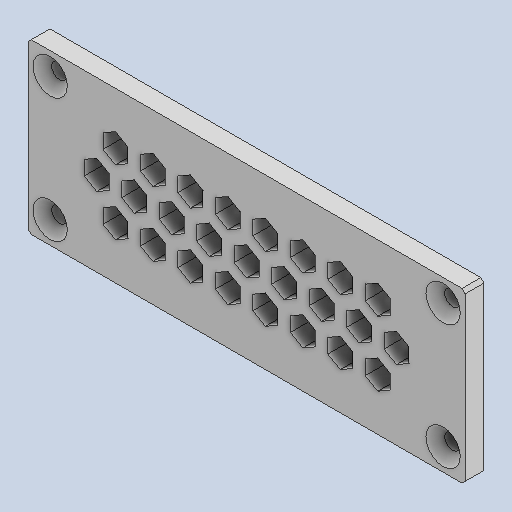
# Autodesk Inventor part: A-04
Saved by Autodesk Inventor 2022.2 (Build 262287000, 287)
## iProperties
Created: 2021-12-13
Part Number: A-04
Material: Generic
Document SubType Name: Modeling
Designer: kfcs7
Density: 1 g/cm^3
Appearance: Default
Author: kfcs7
Autodesk Inventor part; units mm, degrees
ref_plane "YZ Plane" through (0, 0, 0) normal (1, 0, 0) x (0, 1, 0)
ref_plane "XZ Plane" through (0, 0, 0) normal (0, 1, 0) x (-1, 0, 0)
ref_plane "XY Plane" through (0, 0, 0) normal (0, 0, 1) x (1, 0, 0)
sketch "Sketch1" plane through (0, 0, 0) normal (0, 0, 1) x (1, 0, 0)
  circle A0 centre (66.4645, 3.5355) radius 2 construction
  line L0 (0.5, 0) -> (0, 0.5) projected
  line L1 (0.5, 0) -> (69.5, 0) projected
  line L2 (70, 0.5) -> (69.5, 0) projected
  line L3 (70, 0.5) -> (70, 9.5) construction
  line L4 (70, 9.5) -> (67, 9.5) construction
  line L5 (67, 17.5) -> (67, 9.5) construction
  line L6 (65, 17.5) -> (67, 17.5) construction
  line L7 (65, 17.5) -> (65, 8.0711) construction
  line L8 (65, 8.0711) -> (61.9289, 5) construction
  line L9 (61.9289, 5) -> (8.0711, 5) construction
  line L10 (8.0711, 5) -> (5, 8.0711) construction
  line L11 (5, 8.0711) -> (5, 17.5) construction
  line L12 (3, 17.5) -> (5, 17.5) construction
  line L13 (3, 9.5) -> (3, 17.5) construction
  line L14 (3, 9.5) -> (0, 9.5) construction
  line L15 (0, 0.5) -> (0, 9.5) construction
  circle A1 centre (3.5355, 3.5355) radius 2 construction
  circle A2 centre (3.5355, 23.4645) radius 2 construction
  circle A3 centre (66.4645, 23.4645) radius 2 construction
  line L16 (65, 17.5) -> (67.5, 17.5) construction
  line L17 (67.5, 17.5) -> (67.5, 9.5) construction
  line L18 (70, 9.5) -> (67.5, 9.5) construction
  line L19 (70, 26.5) -> (70, 9.5) construction
  line L20 (69.5, 27) -> (70, 26.5) projected
  line L21 (69.5, 27) -> (0.5, 27) projected
  line L22 (0, 26.5) -> (0.5, 27) projected
  line L23 (0, 26.5) -> (0, 9.5) construction
  line L24 (2.5, 9.5) -> (0, 9.5) construction
  line L25 (2.5, 9.5) -> (2.5, 17.5) construction
  line L26 (2.5, 17.5) -> (5, 17.5) construction
  line L27 (5, 17.5) -> (5, 18.9289) construction
  line L28 (5, 18.9289) -> (8.0711, 22) construction
  line L29 (8.0711, 22) -> (61.9289, 22) construction
  line L30 (61.9289, 22) -> (65, 18.9289) construction
  line L31 (65, 18.9289) -> (65, 17.5) construction
  line L32 (70, 26.5) -> (70, 0.5)
  line L33 (0, 0.5) -> (0, 26.5)
  point P0 (0, 0)
  constraints: 4 end point, 2 collinear
extrude "Extrusion1" add sketch "Sketch1" along normal blind 3
sketch "Sketch2" plane through (0, 0, 3) normal (0, 0, 1) x (1, 0, 0)
  circle A0 centre (3.5355, 23.4645) radius 2 construction
  circle A1 centre (66.4645, 23.4645) radius 2 construction
  line L0 (65, 17.5) -> (67.5, 17.5) construction
  line L1 (67.5, 17.5) -> (67.5, 9.5) construction
  line L2 (70, 9.5) -> (67.5, 9.5) construction
  line L3 (70, 26.5) -> (70, 9.5) construction
  line L4 (69.5, 27) -> (70, 26.5) construction
  line L5 (69.5, 27) -> (0.5, 27) construction
  line L6 (0, 26.5) -> (0.5, 27) construction
  line L7 (0, 26.5) -> (0, 9.5) construction
  line L8 (2.5, 9.5) -> (0, 9.5) construction
  line L9 (2.5, 9.5) -> (2.5, 17.5) construction
  line L10 (2.5, 17.5) -> (5, 17.5) construction
  line L11 (5, 17.5) -> (5, 18.9289) construction
  line L12 (5, 18.9289) -> (8.0711, 22) construction
  line L13 (8.0711, 22) -> (61.9289, 22) construction
  line L14 (61.9289, 22) -> (65, 18.9289) construction
  line L15 (65, 18.9289) -> (65, 17.5) construction
  circle A2 centre (66.4645, 3.5355) radius 2 construction
  line L16 (0.5, 0) -> (0, 0.5) construction
  line L17 (0.5, 0) -> (69.5, 0) construction
  line L18 (70, 0.5) -> (69.5, 0) construction
  line L19 (70, 0.5) -> (70, 9.5) construction
  line L20 (70, 9.5) -> (67, 9.5) construction
  line L21 (67, 17.5) -> (67, 9.5) construction
  line L22 (65, 17.5) -> (67, 17.5) construction
  line L23 (65, 17.5) -> (65, 8.0711) construction
  line L24 (65, 8.0711) -> (61.9289, 5) construction
  line L25 (61.9289, 5) -> (8.0711, 5) construction
  line L26 (8.0711, 5) -> (5, 8.0711) construction
  line L27 (5, 8.0711) -> (5, 17.5) construction
  line L28 (3, 17.5) -> (5, 17.5) construction
  line L29 (3, 9.5) -> (3, 17.5) construction
  line L30 (3, 9.5) -> (0, 9.5) construction
  line L31 (0, 0.5) -> (0, 9.5) construction
  circle A3 centre (3.5355, 3.5355) radius 2 construction
  circle A4 centre (3.5355, 23.4645) radius 1.25
  circle A5 centre (3.5355, 3.5355) radius 1.25
  circle A6 centre (66.4645, 3.5355) radius 1.25
  circle A7 centre (66.4645, 23.4645) radius 1.25
  point P0 (0, 0)
  dimension "d2" = 2.5
  dimension "d3" = 2.5
  dimension "d4" = 2.5
  dimension "d5" = 2.5
  constraints: 4 centre point, 4 coincident
  measures "d2" diameter of A4
  measures "d3" diameter of A5
  measures "d4" diameter of A6
  measures "d5" diameter of A7
extrude "Extrusion2" cut sketch "Sketch2" against normal through all
chamfer "Chamfer1" distance 1.5 angle 45 4 edges at (2.2855, 23.4645, 3) (2.2855, 3.5355, 3) (65.2145, 3.5355, 3) (65.2145, 23.4645, 3)
sketch "Sketch3" plane through (0, 0, 3) normal (0, 0, 1) x (1, 0, 0)
  circle A0 centre (66.4645, 3.5355) radius 2.75 projected
  circle A1 centre (3.5355, 23.4645) radius 2.75 projected
  line L0 (0.5, 27) -> (0, 26.5) projected
  line L1 (0, 26.5) -> (0, 0.5) projected
  line L2 (0, 0.5) -> (0.5, 0) projected
  line L3 (0.5, 0) -> (69.5, 0) projected
  line L4 (69.5, 0) -> (70, 0.5) projected
  line L5 (70, 0.5) -> (70, 26.5) projected
  line L6 (70, 26.5) -> (69.5, 27) projected
  line L7 (69.5, 27) -> (0.5, 27) projected
  circle A2 centre (3.5355, 3.5355) radius 2.75 projected
  circle A3 centre (66.4645, 23.4645) radius 2.75 projected
  line L8 (32, 15.2321) -> (35, 16.9641)
  line L9 (35, 16.9641) -> (38, 15.2321)
  line L10 (38, 15.2321) -> (38, 11.7679)
  line L11 (38, 11.7679) -> (35, 10.0359)
  line L12 (35, 10.0359) -> (32, 11.7679)
  line L13 (32, 11.7679) -> (32, 15.2321)
  line L14 (69.5, 27) -> (0.5, 27) projected
  line L15 (35, 15.8094) -> (33, 14.6547)
  line L16 (33, 14.6547) -> (33, 12.3453)
  line L17 (33, 12.3453) -> (35, 11.1906)
  line L18 (35, 11.1906) -> (37, 12.3453)
  line L19 (37, 12.3453) -> (37, 14.6547)
  line L20 (37, 14.6547) -> (35, 15.8094)
  line L21 (35, 16.9641) -> (35, 20.4282)
  line L22 (35, 20.4282) -> (32, 22.1603)
  line L23 (32, 22.1603) -> (29, 20.4282)
  line L24 (29, 20.4282) -> (29, 16.9641)
  line L25 (29, 16.9641) -> (32, 15.2321)
  line L26 (34, 17.5415) -> (32, 16.3868)
  line L27 (32, 16.3868) -> (30, 17.5415)
  line L28 (30, 17.5415) -> (30, 19.8509)
  line L29 (30, 19.8509) -> (32, 21.0056)
  line L30 (32, 21.0056) -> (34, 19.8509)
  line L31 (34, 19.8509) -> (34, 17.5415)
  line L32 (38, 4.8397) -> (41, 6.5718)
  line L33 (41, 6.5718) -> (41, 10.0359)
  line L34 (41, 10.0359) -> (38, 11.7679)
  line L35 (35, 10.0359) -> (35, 6.5718)
  line L36 (35, 6.5718) -> (38, 4.8397)
  line L37 (40, 7.1491) -> (38, 5.9944)
  line L38 (38, 5.9944) -> (36, 7.1491)
  line L39 (36, 7.1491) -> (36, 9.4585)
  line L40 (36, 9.4585) -> (38, 10.6132)
  line L41 (38, 10.6132) -> (40, 9.4585)
  line L42 (40, 9.4585) -> (40, 7.1491)
  point P0 (0, 0)
  point P1 (35, 13.5)
  point P2 (32, 18.6962)
  point P3 (38, 8.3038)
  dimension "d12" = 27
  dimension "d13" = 13.5
  dimension "d14" = 35
  dimension "d15" = 70
  dimension "d16" = 6
  dimension "d19" = 1
  constraints: 68 end point, 22 symmetric about line, 1 perpendicular, 18 other
  measures "d12" distance between parallel lines of L7 L3
  measures "d13" distance from line of L3 point (35, 13.5)
  measures "d14" distance from line of L5 point (35, 13.5)
  measures "d15" distance between parallel lines of L5 L1
  measures "d16" distance between parallel lines of L10 L13
  measures "d19" distance between parallel lines of L8 L15
extrude "Extrusion3" cut sketch "Sketch3" against normal through all contours L20 L19 L18 L17 L16 L15 | L26 L27 L28 L29 L30 L31 | L37 L38 L39 L40 L41 L42
pattern_linear "Rectangular Pattern1" count 9 spacing 6 along (-1, 0, 0) of "Extrusion3" first direction both ways yes
sketch "Sketch4" plane through (0, 0, 3) normal (0, 0, 1) x (1, 0, 0)
  line L0 (16, 7.1491) -> (14, 5.9944) projected
  line L1 (14, 5.9944) -> (12, 7.1491) projected
  line L2 (12, 7.1491) -> (12, 9.4585) projected
  line L3 (12, 9.4585) -> (14, 10.6132) projected
  line L4 (14, 10.6132) -> (16, 9.4585) projected
  line L5 (16, 9.4585) -> (16, 7.1491) projected
  line L6 (11, 15.8094) -> (13, 14.6547) projected
  line L7 (13, 14.6547) -> (13, 12.3453) projected
  line L8 (13, 12.3453) -> (11, 11.1906) projected
  line L9 (11, 11.1906) -> (9, 12.3453) projected
  line L10 (9, 12.3453) -> (9, 14.6547) projected
  line L11 (9, 14.6547) -> (11, 15.8094) projected
  line L12 (6, 17.5415) -> (6, 19.8509) projected
  line L13 (6, 19.8509) -> (8, 21.0056) projected
  line L14 (8, 21.0056) -> (10, 19.8509) projected
  line L15 (10, 19.8509) -> (10, 17.5415) projected
  line L16 (10, 17.5415) -> (8, 16.3868) projected
  line L17 (8, 16.3868) -> (6, 17.5415) projected
  line L18 (22, 7.1491) -> (20, 5.9944) projected
  line L19 (20, 5.9944) -> (18, 7.1491) projected
  line L20 (18, 7.1491) -> (18, 9.4585) projected
  line L21 (18, 9.4585) -> (20, 10.6132) projected
  line L22 (20, 10.6132) -> (22, 9.4585) projected
  line L23 (22, 9.4585) -> (22, 7.1491) projected
  line L24 (17, 15.8094) -> (19, 14.6547) projected
  line L25 (19, 14.6547) -> (19, 12.3453) projected
  line L26 (19, 12.3453) -> (17, 11.1906) projected
  line L27 (17, 11.1906) -> (15, 12.3453) projected
  line L28 (15, 12.3453) -> (15, 14.6547) projected
  line L29 (15, 14.6547) -> (17, 15.8094) projected
  line L30 (12, 17.5415) -> (12, 19.8509) projected
  line L31 (12, 19.8509) -> (14, 21.0056) projected
  line L32 (14, 21.0056) -> (16, 19.8509) projected
  line L33 (16, 19.8509) -> (16, 17.5415) projected
  line L34 (16, 17.5415) -> (14, 16.3868) projected
  line L35 (14, 16.3868) -> (12, 17.5415) projected
  line L36 (28, 7.1491) -> (26, 5.9944) projected
  line L37 (26, 5.9944) -> (24, 7.1491) projected
  line L38 (24, 7.1491) -> (24, 9.4585) projected
  line L39 (24, 9.4585) -> (26, 10.6132) projected
  line L40 (26, 10.6132) -> (28, 9.4585) projected
  line L41 (28, 9.4585) -> (28, 7.1491) projected
  line L42 (23, 15.8094) -> (25, 14.6547) projected
  line L43 (25, 14.6547) -> (25, 12.3453) projected
  line L44 (25, 12.3453) -> (23, 11.1906) projected
  line L45 (23, 11.1906) -> (21, 12.3453) projected
  line L46 (21, 12.3453) -> (21, 14.6547) projected
  line L47 (21, 14.6547) -> (23, 15.8094) projected
  line L48 (18, 17.5415) -> (18, 19.8509) projected
  line L49 (18, 19.8509) -> (20, 21.0056) projected
  line L50 (20, 21.0056) -> (22, 19.8509) projected
  line L51 (22, 19.8509) -> (22, 17.5415) projected
  line L52 (22, 17.5415) -> (20, 16.3868) projected
  line L53 (20, 16.3868) -> (18, 17.5415) projected
  line L54 (34, 7.1491) -> (32, 5.9944) projected
  line L55 (32, 5.9944) -> (30, 7.1491) projected
  line L56 (30, 7.1491) -> (30, 9.4585) projected
  line L57 (30, 9.4585) -> (32, 10.6132) projected
  line L58 (32, 10.6132) -> (34, 9.4585) projected
  line L59 (34, 9.4585) -> (34, 7.1491) projected
  line L60 (29, 15.8094) -> (31, 14.6547) projected
  line L61 (31, 14.6547) -> (31, 12.3453) projected
  line L62 (31, 12.3453) -> (29, 11.1906) projected
  line L63 (29, 11.1906) -> (27, 12.3453) projected
  line L64 (27, 12.3453) -> (27, 14.6547) projected
  line L65 (27, 14.6547) -> (29, 15.8094) projected
  line L66 (24, 17.5415) -> (24, 19.8509) projected
  line L67 (24, 19.8509) -> (26, 21.0056) projected
  line L68 (26, 21.0056) -> (28, 19.8509) projected
  line L69 (28, 19.8509) -> (28, 17.5415) projected
  line L70 (28, 17.5415) -> (26, 16.3868) projected
  line L71 (26, 16.3868) -> (24, 17.5415) projected
  line L72 (46, 7.1491) -> (44, 5.9944) projected
  line L73 (44, 5.9944) -> (42, 7.1491) projected
  line L74 (42, 7.1491) -> (42, 9.4585) projected
  line L75 (42, 9.4585) -> (44, 10.6132) projected
  line L76 (44, 10.6132) -> (46, 9.4585) projected
  line L77 (46, 9.4585) -> (46, 7.1491) projected
  line L78 (41, 15.8094) -> (43, 14.6547) projected
  line L79 (43, 14.6547) -> (43, 12.3453) projected
  line L80 (43, 12.3453) -> (41, 11.1906) projected
  line L81 (41, 11.1906) -> (39, 12.3453) projected
  line L82 (39, 12.3453) -> (39, 14.6547) projected
  line L83 (39, 14.6547) -> (41, 15.8094) projected
  line L84 (36, 17.5415) -> (36, 19.8509) projected
  line L85 (36, 19.8509) -> (38, 21.0056) projected
  line L86 (38, 21.0056) -> (40, 19.8509) projected
  line L87 (40, 19.8509) -> (40, 17.5415) projected
  line L88 (40, 17.5415) -> (38, 16.3868) projected
  line L89 (38, 16.3868) -> (36, 17.5415) projected
  line L90 (52, 7.1491) -> (50, 5.9944) projected
  line L91 (50, 5.9944) -> (48, 7.1491) projected
  line L92 (48, 7.1491) -> (48, 9.4585) projected
  line L93 (48, 9.4585) -> (50, 10.6132) projected
  line L94 (50, 10.6132) -> (52, 9.4585) projected
  line L95 (52, 9.4585) -> (52, 7.1491) projected
  line L96 (47, 15.8094) -> (49, 14.6547) projected
  line L97 (49, 14.6547) -> (49, 12.3453) projected
  line L98 (49, 12.3453) -> (47, 11.1906) projected
  line L99 (47, 11.1906) -> (45, 12.3453) projected
  line L100 (45, 12.3453) -> (45, 14.6547) projected
  line L101 (45, 14.6547) -> (47, 15.8094) projected
  line L102 (42, 17.5415) -> (42, 19.8509) projected
  line L103 (42, 19.8509) -> (44, 21.0056) projected
  line L104 (44, 21.0056) -> (46, 19.8509) projected
  line L105 (46, 19.8509) -> (46, 17.5415) projected
  line L106 (46, 17.5415) -> (44, 16.3868) projected
  line L107 (44, 16.3868) -> (42, 17.5415) projected
  line L108 (58, 7.1491) -> (56, 5.9944) projected
  line L109 (56, 5.9944) -> (54, 7.1491) projected
  line L110 (54, 7.1491) -> (54, 9.4585) projected
  line L111 (54, 9.4585) -> (56, 10.6132) projected
  line L112 (56, 10.6132) -> (58, 9.4585) projected
  line L113 (58, 9.4585) -> (58, 7.1491) projected
  line L114 (53, 15.8094) -> (55, 14.6547) projected
  line L115 (55, 14.6547) -> (55, 12.3453) projected
  line L116 (55, 12.3453) -> (53, 11.1906) projected
  line L117 (53, 11.1906) -> (51, 12.3453) projected
  line L118 (51, 12.3453) -> (51, 14.6547) projected
  line L119 (51, 14.6547) -> (53, 15.8094) projected
  line L120 (48, 17.5415) -> (48, 19.8509) projected
  line L121 (48, 19.8509) -> (50, 21.0056) projected
  line L122 (50, 21.0056) -> (52, 19.8509) projected
  line L123 (52, 19.8509) -> (52, 17.5415) projected
  line L124 (52, 17.5415) -> (50, 16.3868) projected
  line L125 (50, 16.3868) -> (48, 17.5415) projected
  line L126 (64, 7.1491) -> (62, 5.9944) projected
  line L127 (62, 5.9944) -> (60, 7.1491) projected
  line L128 (60, 7.1491) -> (60, 9.4585) projected
  line L129 (60, 9.4585) -> (62, 10.6132) projected
  line L130 (62, 10.6132) -> (64, 9.4585) projected
  line L131 (64, 9.4585) -> (64, 7.1491) projected
  line L132 (59, 15.8094) -> (61, 14.6547) projected
  line L133 (61, 14.6547) -> (61, 12.3453) projected
  line L134 (61, 12.3453) -> (59, 11.1906) projected
  line L135 (59, 11.1906) -> (57, 12.3453) projected
  line L136 (57, 12.3453) -> (57, 14.6547) projected
  line L137 (57, 14.6547) -> (59, 15.8094) projected
  line L138 (54, 17.5415) -> (54, 19.8509) projected
  line L139 (54, 19.8509) -> (56, 21.0056) projected
  line L140 (56, 21.0056) -> (58, 19.8509) projected
  line L141 (58, 19.8509) -> (58, 17.5415) projected
  line L142 (58, 17.5415) -> (56, 16.3868) projected
  line L143 (56, 16.3868) -> (54, 17.5415) projected
  line L144 (36, 9.4585) -> (38, 10.6132) projected
  line L145 (38, 10.6132) -> (40, 9.4585) projected
  line L146 (40, 9.4585) -> (40, 7.1491) projected
  line L147 (40, 7.1491) -> (38, 5.9944) projected
  line L148 (38, 5.9944) -> (36, 7.1491) projected
  line L149 (36, 7.1491) -> (36, 9.4585) projected
  line L150 (32, 21.0056) -> (34, 19.8509) projected
  line L151 (34, 19.8509) -> (34, 17.5415) projected
  line L152 (34, 17.5415) -> (32, 16.3868) projected
  line L153 (32, 16.3868) -> (30, 17.5415) projected
  line L154 (30, 17.5415) -> (30, 19.8509) projected
  line L155 (30, 19.8509) -> (32, 21.0056) projected
  line L156 (35, 11.1906) -> (33, 12.3453) projected
  line L157 (33, 12.3453) -> (33, 14.6547) projected
  line L158 (33, 14.6547) -> (35, 15.8094) projected
  line L159 (35, 15.8094) -> (37, 14.6547) projected
  line L160 (37, 14.6547) -> (37, 12.3453) projected
  line L161 (37, 12.3453) -> (35, 11.1906) projected
  circle A0 centre (66.4645, 3.5355) radius 2.75 projected
  circle A1 centre (3.5355, 23.4645) radius 2.75 projected
  line L162 (0.5, 27) -> (0, 26.5) projected
  line L163 (0, 26.5) -> (0, 0.5) projected
  line L164 (0, 0.5) -> (0.5, 0) projected
  line L165 (0.5, 0) -> (69.5, 0) projected
  line L166 (69.5, 0) -> (70, 0.5) projected
  line L167 (70, 0.5) -> (70, 26.5) projected
  line L168 (70, 26.5) -> (69.5, 27) projected
  line L169 (69.5, 27) -> (0.5, 27) projected
  circle A2 centre (3.5355, 3.5355) radius 2.75 projected
  circle A3 centre (66.4645, 23.4645) radius 2.75 projected
  point P0 (0, 0)
extrude "Extrusion4" add sketch "Sketch4" against normal up to surface (3 mm away) contours L12 L13 L14 L15 L16 L17 | L126 L127 L128 L129 L130 L131
equation "\"d3\" = d2"
equation "\"d4\" = d2"
equation "\"d5\" = d2"
equation "\"d13\" = 0.5 * d12"
equation "\"d14\" = 0.5 * d15"
body "Solid1"
